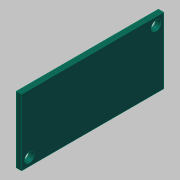
# Autodesk Inventor part: Parallax_Ping_PCB
Saved by Autodesk Inventor 2012 (Build 160160000, 160)
## iProperties
Manager: Ed Sparks
Company: FirstCadLibrary
Shininess: 64.0
Length Units: 11269
Angle Units: 11279
Time Units: 11290
Mass Units: 11283
Length Display Precision: 3
Angle Display Precision: 2
Compacted: True
Part Number: Parallax_Ping_PCB
Document SubType Name: Modeling
Created: 2007-01-24
Designer: Ed Sparks
Material: Phenolic
Catalog Web Link: www.firstcadlibrary.com
Engineer: Ed Sparks
Density: 1.38 g/cm^3
Mass: 2.31433 g
Surface Area: 21.8522 cm^2
Volume: 1.67705 cm^3
Density: 0.0
Volumn: 0.0
Area: 0.0
PropertySet Name: Model Information
Control State: 0
Master: False
Checked Out: False
Author: Ed Sparks
Keywords: FIRST
Autodesk Inventor part; units mm, degrees
ref_plane "YZ Plane" through (0, 0, 0) normal (1, 0, 0) x (0, 1, 0)
ref_plane "XZ Plane" through (0, 0, 0) normal (0, 1, 0) x (-1, 0, 0)
ref_plane "XY Plane" through (0, 0, 0) normal (0, 0, 1) x (1, 0, 0)
sketch "Sketch1" plane through (0, 0, 0) normal (0, 0, 1) x (1, 0, 0)
  line L0 (-22.85, 10.65) -> (22.85, 10.65)
  line L1 (22.85, 10.65) -> (22.85, -10.65)
  line L2 (22.85, -10.65) -> (-22.85, -10.65)
  line L3 (-22.85, -10.65) -> (-22.85, 10.65)
  line L4 (0, 0) -> (0, 10.65) construction
  line L5 (0, 0) -> (0, -10.65) construction
  line L6 (0, 0) -> (22.85, 0) construction
  line L7 (0, 0) -> (-22.85, 0) construction
  dimension "d0" = 45.7
  dimension "d1" = 21.3
  constraints: 16 end point, 4 midpoint, 2 collinear, 2 parallel, 1 horizontal, 1 perpendicular, 1 other
  measures "d0" distance of L0.start L0.end
  measures "d1" distance of L2.end L0.start
extrude "Extrusion1" add sketch "Sketch1" along normal blind 1.75
sketch "Sketch2" plane through (0, 0, 1.75) normal (0, 0, 1) x (1, 0, 0)
  line L0 (22.85, 10.65) -> (22.85, -10.65) projected
  line L1 (-22.85, 10.65) -> (22.85, 10.65) projected
  line L2 (22.85, -10.65) -> (-22.85, -10.65) projected
  point P0 (-20.35, -8.15)
  point P1 (20.35, 8.15)
  dimension "d4" = 2.5
  dimension "d5" = 2.5
  dimension "d6" = 2.5
  dimension "d7" = 2.5
  measures "d4" horizontal distance of point (-20.35, -8.15) L2.end
  measures "d5" distance from line of L2 point (-20.35, -8.15)
  measures "d6" distance from line of L0 point (20.35, 8.15)
  measures "d7" distance from line of L1 point (20.35, 8.15)
hole "Hole1" at (-20.35, -8.15, 1.75) at (20.35, 8.15, 1.75) direction (0, 0, -1) diameter 3.1 end through all
body "Solid1"
